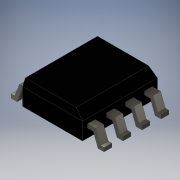
# Autodesk Inventor part: MC34063
Saved by Autodesk Inventor 2016 (Build 200138000, 138)
## iProperties
Created: 2016-08-10
Part Number: MC34063
Material: Generic
Document SubType Name: Modeling
Designer: jfixelle
Density: 1 g/cm^3
Appearance: Black
Author: jfixelle
Autodesk Inventor part; units mm, degrees
ref_plane "YZ Plane" through (0, 0, 0) normal (1, 0, 0) x (0, 1, 0)
ref_plane "XZ Plane" through (0, 0, 0) normal (0, 1, 0) x (-1, 0, 0)
sketch "Sketch1" plane through (0, 0, 0) normal (0, 1, 0) x (-1, 0, 0)
  line L0 (2, 2.5) -> (-2, 2.5)
  line L1 (-2, 2.5) -> (-2, -2.5)
  line L2 (-2, -2.5) -> (2, -2.5)
  line L3 (2, -2.5) -> (2, 2.5)
  point P0 (0, 0)
  dimension "d0" = 4
  dimension "d1" = 5
  dimension "d2" = 2
  dimension "d3" = 2.5
  constraints: 8 end point, 2 parallel, 1 horizontal, 1 perpendicular
  measures "d0" distance of L1.end L2.end
  measures "d1" distance of L2.end L0.start
  measures "d2" distance from line of L3 point (0, 0)
  measures "d3" distance from line of point (0, 0) L2
extrude "Extrusion1" add sketch "Sketch1" along normal blind 1.65
chamfer "Chamfer1" distance 0.5 angle 10 1 edges at (0, 1.65, 2.5) measured on face at (-0.6667, 0.55, 2.5)
chamfer "Chamfer2" distance 0.5 angle 10 1 edges at (-2, 1.65, -0.0441) measured on face at (-2, 0.9333, -0.8333)
chamfer "Chamfer3" distance 0.5 angle 10 1 edges at (0.0441, 1.65, -2.5) measured on face at (0.6667, 0.9333, -2.5)
chamfer "Chamfer4" distance 0.5 angle 45 1 edges at (2, 1.65, 0) measured on face at (2, 0.3833, 0.8333)
ref_plane "Work Plane1" through (2, 0, -1.905) normal (0, 0, -1) x (-1, 0, 0)
sketch "Sketch2" plane through (2, 0, -1.905) normal (0, 0, -1) x (-1, 0, 0)
  line L0 (0, 0.825) -> (0, 0.575)
  line L1 (0, 0.575) -> (-0.3809, 0.575)
  line L2 (-0.3809, 0.575) -> (-0.7, -0.25)
  line L3 (-0.7, -0.25) -> (-1.1, -0.25)
  line L4 (-1.1, -0.25) -> (-1.1, 0)
  line L5 (-1.1, 0) -> (-0.8681, 0)
  line L6 (-0.8681, 0) -> (-0.549, 0.825)
  line L7 (-0.549, 0.825) -> (0, 0.825)
  line L8 (0, 0) -> (0, 1.15) projected
  line L9 (0, 0) -> (4, 0) projected
  point P0 (2, 0)
  dimension "d19" = 0
  dimension "d20" = 0.25
  dimension "d21" = 0.25
  dimension "d22" = 0.4
  dimension "d23" = 1.1
  dimension "d24" = 0.25
  dimension "d25" = 0.825
  constraints: 16 end point, 3 parallel, 3 perpendicular, 1 vertical
  measures "d19" distance between parallel lines of L0 L8
  measures "d20" distance between parallel lines of L1 L7
  measures "d21" distance of L3.end L4.end
  measures "d22" distance of L3.end L2.end
  measures "d23" distance between parallel lines of L0 L4
  measures "d24" distance between parallel lines of L9 L3
  measures "d25" distance between parallel lines of L9 L7
extrude "Extrusion2" add sketch "Sketch2" along normal mid plane 0.51
pattern_linear "Rectangular Pattern1" count 4 spacing 1.27 along (0, 0, 1) of "Extrusion2"
mirror "Mirror1" about plane through (0, 0, 0) normal (1, 0, 0) of "Extrusion2", "Rectangular Pattern1"
body "Solid1"
